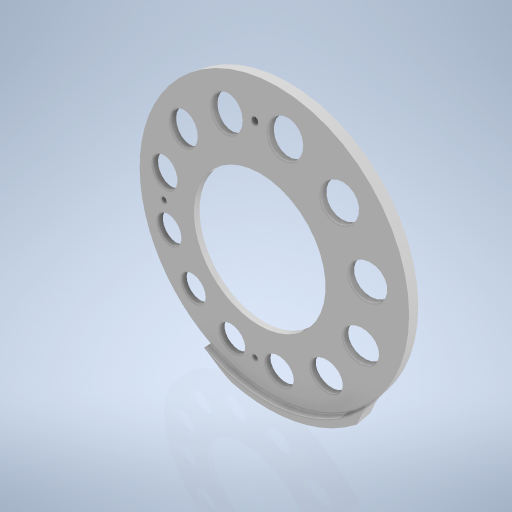
# Autodesk Inventor part: nockenscheibe2
Saved by Autodesk Inventor 2024.2 (Build 282272000, 272)
## iProperties
Created: 2024-04-30
Part Number: nockenscheibe2
Material: Generisch
Document SubType Name: Modeling
Designer: Fabri
Density: 1 g/cm^3
Appearance: Vorgabe
Author: Fabri
Autodesk Inventor part; units mm, degrees
ref_plane "YZ Plane" through (0, 0, 0) normal (1, 0, 0) x (0, 1, 0)
ref_plane "XZ Plane" through (0, 0, 0) normal (0, 1, 0) x (-1, 0, 0)
ref_plane "XY Plane" through (0, 0, 0) normal (0, 0, 1) x (1, 0, 0)
sketch "Skizze1" plane through (0, 0, 0) normal (0, 1, 0) x (-1, 0, 0)
  circle A0 centre (0, 0) radius 35
  dimension "d7" = 70
  constraints: 1 centre point, 1 coincident
  measures "d7" diameter of A0
extrude "Extrusion1" add sketch "Skizze1" along normal blind 2.5
sketch "Skizze3" plane through (0, 2.5, 0) normal (0, 1, 0) x (1, 0, 0)
  circle A0 centre (0, 0) radius 35 projected
  constraints: 1 coincident
hole "Bohrung1" at (0, 2.5, 0) direction (0, -1, 0) diameter 35 depth 2.5 counterbore diameter 69 counterbore depth 1
sketch "Skizze4" plane through (0, 0, 0) normal (0, -1, 0) x (1, 0, 0)
  circle A0 centre (0, 0) radius 27 construction
  line L0 (0, 0) -> (-42.7199, -11.4468) construction
  line L1 (0, 0) -> (-46.622, 0) construction
  line L2 (0, 0) -> (-37.3681, 21.5745) construction
  point P0 (-26.08, -6.9881)
  dimension "d25" = 54
  dimension "d26" = 15
  dimension "d27" = 30
  dimension "d28" = 45
  constraints: 6 end point, 1 coincident, 1 horizontal, 1 point on line, 3 other
  measures "d26" angle of L0 L1
  measures "d27" angle of L1 L2
  measures "d28" angle of L0 L2
hole "Bohrung2" at (-26.08, 0, -6.9881) direction (0, 1, 0) diameter 8 end through all
pattern_circular "Runde Anordnung1" count 12 over 360 about axis through (0, -96.5265, 0) along (0, 1, 0) of "Bohrung2"
sketch "Skizze5" plane through (0, 0, 0) normal (0, -1, 0) x (1, 0, 0)
  circle A0 centre (0, 0) radius 27 construction
  line L0 (0, 0) -> (-37.3681, 21.5745) construction
  line L1 (0, 0) -> (-46.622, 0) construction
  circle A1 centre (0, 0) radius 35 projected
  line L2 (0, 0) -> (-42.7199, -11.4468) construction
  point P0 (0, -27)
  point P1 (0, 27)
  point P2 (-27, 0)
  constraints: 3 point on circle, 2 vertical alignment, 1 point on line
hole "Bohrung3" at (0, 0, -27) at (-27, 0, 0) at (0, 0, 27) direction (0, 1, 0) diameter 1.567 depth 1.5 thread size "M2x0.4" class "6H" standard "ISO Metric profile"
sketch "Skizze6" plane through (0, 0, 0) normal (0, -1, 0) x (1, 0, 0)
  arc A0 (-5.2244, -36.6293) -> (28.4893, -23.6085) centre (0, 0) ccw
  circle A1 centre (0, 0) radius 35 projected
  arc A2 (-10.7196, -33.956) -> (-14.1572, -32.0089) centre (-22.2471, -50.2998) ccw
  arc A3 (-10.7196, -33.956) -> (-5.2244, -36.6293) centre (0.2314, -18.4295) ccw
  arc A4 (28.4893, -23.6085) -> (28.8475, -22.117) centre (10.2088, -18.4295) ccw
  arc A5 (30.8428, -16.5446) -> (28.8475, -22.117) centre (48.4672, -25.9987) ccw
  dimension "d39" = 74
  dimension "d56" = 20
  dimension "d57" = 19
  dimension "d58" = 19
  dimension "d59" = 20
  dimension "d60" = 45
  constraints: 12 point on circle, 5 centre point, 4 tangent, 1 coincident, 1 horizontal alignment
  measures "d39" diameter of A0
  measures "d56" radius of A2
  measures "d57" radius of A3
  measures "d58" radius of A4
  measures "d59" radius of A5
  measures "d60" horizontal distance of A1.end A1.start
extrude "Extrusion2" add sketch "Skizze6" along normal mid plane 4 contours A3 A2 A1 A5 A4 A0
